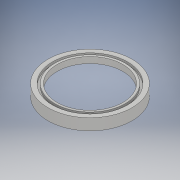
# Autodesk Inventor part: Shaft
Saved by Autodesk Inventor 2018 (Build 220112000, 112)
## iProperties
Created: 2017-06-25
Part Number: Shaft
Material: Generic
Document SubType Name: Modeling
Designer: Soichi
Density: 1 g/cm^3
Appearance: Default
Author: Soichi
Autodesk Inventor part; units mm, degrees
ref_plane "YZ Plane" through (0, 0, 0) normal (1, 0, 0) x (0, 1, 0)
ref_plane "XZ Plane" through (0, 0, 0) normal (0, 1, 0) x (-1, 0, 0)
ref_plane "XY Plane" through (0, 0, 0) normal (0, 0, 1) x (1, 0, 0)
sketch "Sketch3" plane through (0, 0, 0) normal (0, 0, 1) x (1, 0, 0)
  circle A0 centre (0, 0) radius 55.5
  dimension "d5" = 111
  constraints: 1 centre point, 1 coincident
  measures "d5" diameter of A0
sketch "Sketch4" plane through (0, 0, 0) normal (1, 0, 0) x (0, 1, 0)
  line L0 (55.5, 0) -> (-55.5, 0) construction
  line L1 (-55.5, 0) -> (-55.5, 15)
  line L2 (-55.5, 0) -> (-40.5, 0) construction
  line L3 (-55.5, 0) -> (-49.5, 0) construction
  line L4 (-49.5, 0) -> (-49.5, 3.5)
  line L5 (-49.5, 3.5) -> (-46.42, 3.5)
  line L6 (-49.5, 3.5) -> (-46.42, 3.5) construction
  line L7 (-46.42, 3.5) -> (-46.42, 0)
  line L8 (-46.42, 3.5) -> (-42.92, 3.5) construction
  line L9 (-46.42, 0) -> (-43.5, 0)
  line L10 (-43.5, 0) -> (-43.5, 8)
  line L11 (-43.5, 8) -> (-55.5, 15)
  line L12 (-55.5, 0) -> (-49.5, 0)
  line L13 (-49.5, 0) -> (-49.5, 3.5)
  line L14 (-43.5, 0) -> (-43.5, 8)
  line L15 (-43.5, 8) -> (-55.5, 15)
  line L16 (-55.5, 0) -> (-49.5, 0)
  line L17 (-49.5, 0) -> (-49.5, 3.5)
  line L18 (-46.42, 3.5) -> (-49.5, 3.5)
  line L19 (-46.42, 3.5) -> (-46.42, 0)
  line L20 (-46.42, 0) -> (-43.5, 0)
  point P0 (0, 0)
  dimension "d6" = 15
  dimension "d7" = 90
  dimension "d9" = 3.5
  dimension "d10" = 90
  dimension "d11" = 3.08
  dimension "d12" = 0
  dimension "d13" = 90
  dimension "d15" = 8
  dimension "d18" = 12
  dimension "d19" = 6
  constraints: 40 end point, 6 collinear, 4 horizontal, 3 equal length, 3 perpendicular, 3 point on line, 1 parallel, 1 vertical
  measures "d6" distance of L0.end L1.end
  measures "d7" angle of L2 L1
  measures "d9" distance of L3.end L4.end
  measures "d10" angle of L4 L3
  measures "d11" distance of L4.end L5.end
  measures "d12" distance between parallel lines of L5 L6
  measures "d13" angle of L7 L8
  measures "d15" distance of L9.end L10.end
  measures "d18" distance between parallel lines of L1 L10
  measures "d19" distance between parallel lines of L1 L4
sweep "Sweep1" add profiles "Sketch4" path "Sketch3"
body "Solid2"
